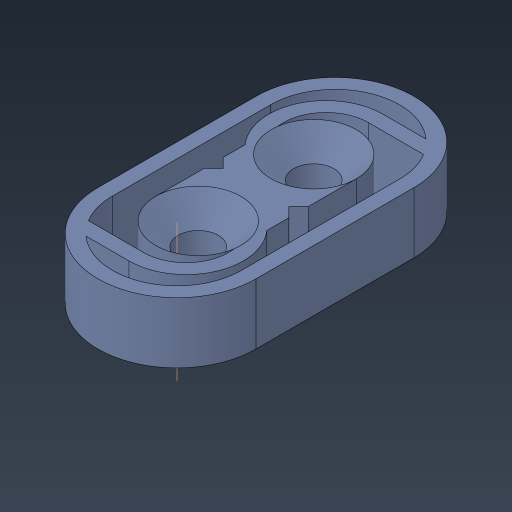
# Autodesk Inventor part: Dribbler Slider v2
Saved by Autodesk Inventor 2023.1 (Build 271208000, 208)
## iProperties
Part Number: Dribbler Slider v2
Material: Gummi, Silikon
Document SubType Name: Modeling
Designer: rYan
Mass: 1.05946 g
Surface Area: 7.33408 cm^2
Volume: 0.847566 cm^3
Density: 1.25 g/cm^3
Appearance: Gummi - Blau
Author: rYan
Autodesk Inventor part; units mm, degrees
ref_plane "YZ Plane" through (0, 0, 0) normal (1, 0, 0) x (0, 1, 0)
ref_plane "XZ Plane" through (0, 0, 0) normal (0, 1, 0) x (-1, 0, 0)
ref_plane "XY Plane" through (0, 0, 0) normal (0, 0, 1) x (1, 0, 0)
sketch "Skizze1" plane through (0, 0, 0) normal (0, 0, 1) x (1, 0, 0)
  line L0 (0, -1.75) -> (0, 11.25) construction
  line L1 (6.5, -1.75) -> (6.5, 11.25)
  line L2 (-6.5, 11.25) -> (-6.5, -1.75)
  arc A0 (-6.5, -1.75) -> (6.5, -1.75) centre (0, -1.75) ccw
  arc A1 (6.5, 11.25) -> (-6.5, 11.25) centre (0, 11.25) ccw
  line L3 (0, 0) -> (0, 9.5) construction
  line L4 (5, -11) -> (-5, -11) construction
  line L5 (0, 0) -> (0, -11) construction
  line L6 (-8.5, 9.1711) -> (-8.5, -11) construction
  point P0 (0, 4.75)
  dimension "d0" = 13
  dimension "d1" = 13
  dimension "d14" = 9.5
  dimension "d17" = 0
  dimension "d26" = 11
  dimension "d27" = 10
  dimension "d28" = 9.25
  dimension "d29" = 8.5
  dimension "d30" = 8.5
  constraints: 16 end point, 4 point on circle, 4 tangent, 3 coincident, 3 midpoint, 3 vertical, 2 centre point, 1 horizontal, 1 parallel, 1 point on line
  measures "d0" diameter of A1
  measures "d1" distance of L0.start L0.end
  measures "d14" distance of L3.start L3.end
  measures "d17" distance between parallel lines of L0 L3
  measures "d26" distance from line of L4 L3.start
  measures "d27" distance of L4.start L4.end
  measures "d28" distance from line of L4 L0.start
  measures "d29" distance between parallel lines of L6 L3
  measures "d30" distance from line of L0.start L6
extrude "Extrusion1" add sketch "Skizze1" against normal blind 5
hole "Bohrung2" at (0, 9.5, 0) at (0, 0, 0) direction (0, 0, -1) diameter 3.3 end through all countersink diameter 7 countersink angle 90
sketch "Skizze5" plane through (0, 0, 0) normal (0, 0, 1) x (1, 0, 0)
  circle A0 centre (0, 9.5) radius 3.5 projected
  circle A1 centre (0, 0) radius 3.5 projected
  line L0 (6.5, -1.75) -> (6.5, 11.25) projected
  arc A2 (6.5, 11.25) -> (-6.5, 11.25) centre (0, 11.25) ccw projected
  line L1 (-6.5, 11.25) -> (-6.5, -1.75) projected
  arc A3 (-6.5, -1.75) -> (6.5, -1.75) centre (0, -1.75) ccw projected
  arc A4 (5.3, 11.25) -> (-5.3, 11.25) centre (0, 11.25) ccw
  line L2 (5.3, 11.25) -> (5.3, -1.75)
  arc A5 (-5.3, -1.75) -> (5.3, -1.75) centre (0, -1.75) ccw
  line L3 (-5.3, -1.75) -> (-5.3, 11.25)
  arc A6 (0, 14) -> (-3.4641, 10) centre (0, 10.5) ccw
  arc A7 (0, 15.2) -> (-3.5, 7.3631) centre (0, 10.5) ccw
  line L4 (-3.5, 9.5) -> (-3.5, 0)
  line L5 (3.5, 9.5) -> (3.5, 0)
  circle A8 centre (0, 9.5) radius 3.5 projected
  circle A9 centre (0, 0) radius 3.5 projected
  line L6 (0, 23.6739) -> (0, -14.1739) construction
  arc A10 (0, -5.7) -> (3.5, 2.1369) centre (0, -1) ccw
  line L7 (0, -4.5) -> (-4.5307, -4.5)
  line L8 (0, -5.7) -> (-3.5338, -5.7)
  line L9 (0, 15.2) -> (3.5338, 15.2)
  line L10 (0, 14) -> (4.5307, 14)
  arc A11 (0, -4.5) -> (3.4641, -0.5) centre (0, -1) ccw
  point P0 (3.5, 2.6665)
  dimension "d47" = 1.2
  dimension "d48" = 1.2
  dimension "d50" = 1
  dimension "d60" = 3.5
  dimension "d61" = 1
  dimension "d62" = 1.2
  dimension "d63" = 3.5
  constraints: 22 point on circle, 16 end point, 6 centre point, 4 tangent, 3 horizontal, 3 point on line, 2 coincident, 1 parallel, 10 other
  measures "d47" radial gap between concentric circles of A2 A4
  measures "d48" radial gap between concentric circles of A7 A6
  measures "d50" distance of A0.centre A6.centre
  measures "d60" radius of A6
  measures "d61" distance of A10.centre point (0, 0)
  measures "d62" radial gap between concentric circles of A11 A10
  measures "d63" radius of A11
extrude "Extrusion4" cut sketch "Skizze5" against normal through all contours A0 A6 L10 A4 L2 A5 L8 A10 L5 | L4 A1 A11 L7 A5 L3 A4 L9 A7
sketch "Skizze6" plane through (0, 0, 0) normal (0, 0, 1) x (1, 0, 0)
  line L0 (-3.5, 7.3631) -> (-3.5, 0) projected
  line L1 (3.5, 2.1369) -> (3.5, 9.5) projected
  circle A0 centre (0, 9.5) radius 1.65 projected
  circle A1 centre (0, 0) radius 1.65 projected
  line L2 (0, 0) -> (0, 9.5) construction
  line L3 (3.5, 4.75) -> (-3.5, 4.75) construction
  line L4 (3.5, 5.55) -> (2.7, 4.75)
  line L5 (3.5, 3.95) -> (2.7, 4.75)
  line L6 (-3.5, 5.55) -> (-2.7, 4.75)
  line L7 (-2.7, 4.75) -> (-3.5, 3.95)
  point P0 (0, 4.75)
  dimension "d64" = 0.8
  constraints: 12 end point, 8 point on line, 2 midpoint, 1 horizontal, 1 parallel, 1 perpendicular, 1 vertical, 2 other
  measures "d64" distance from line of L0 L6.end
extrude "Markierung" cut sketch "Skizze6" against normal through all contours L6 L7 L0 | L5 L4 L1
equation "\"d_Boden\" = 9.5"
equation "\"d_Vorne\" = 9"
equation "\"d_Arm\" = 1.2"
